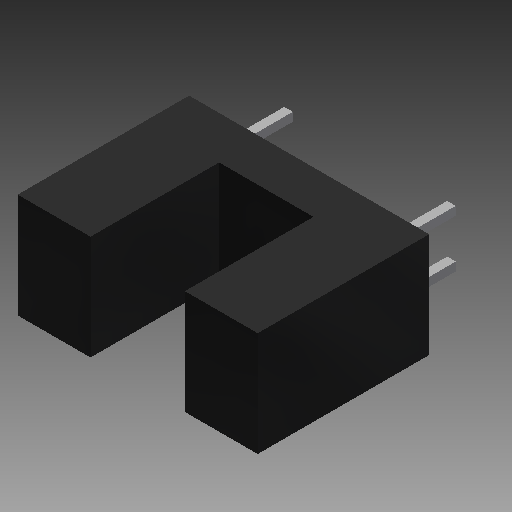
# Autodesk Inventor part: tacometer_ct
Saved by Autodesk Inventor 2019.4 (Build 234330000, 330)
## iProperties
Created: 2019-10-30
Part Number: tacometer_ct
Material: ABS Plastic
Document SubType Name: Modeling
Designer: UFABC
Density: 1 g/cm^3
Appearance: Liso - Branco
Author: UFABC
Autodesk Inventor part; units mm, degrees
ref_plane "YZ Plane" through (0, 0, 0) normal (1, 0, 0) x (0, 1, 0)
ref_plane "XZ Plane" through (0, 0, 0) normal (0, 1, 0) x (-1, 0, 0)
ref_plane "XY Plane" through (0, 0, 0) normal (0, 0, 1) x (1, 0, 0)
sketch "Sketch1" plane through (0, 0, 0) normal (0, 1, 0) x (-1, 0, 0)
  line L0 (-6.3436, 0) -> (7.6564, 0)
  line L1 (7.6564, 0) -> (7.6564, 10)
  line L2 (3.4064, 10) -> (3.4064, 2.5)
  line L3 (3.4064, 2.5) -> (-2.0936, 2.5)
  line L4 (-2.0936, 2.5) -> (-2.0936, 10)
  line L5 (-6.3436, 10) -> (-6.3436, 0)
  line L6 (-6.3436, 10) -> (-2.0936, 10)
  line L7 (3.4064, 10) -> (7.6564, 10)
  point P0 (0, 0)
  dimension "d0" = 10
  dimension "d2" = 14
  dimension "d3" = 2.5
  dimension "d24" = 4.25
  dimension "d25" = 4.25
  constraints: 16 end point, 4 parallel, 2 perpendicular, 1 collinear, 1 horizontal
  measures "d0" distance of L0.end L1.end
  measures "d2" distance of L0.start L0.end
  measures "d3" distance between parallel lines of L0 L3
  measures "d24" distance of L5.start L4.end
  measures "d25" distance of L2.start L1.end
extrude "Extrusion1" add sketch "Sketch1" along normal blind 6.1
sketch "Sketch2" plane through (6.3436, 0, 0) normal (0, 0, -1) x (-1, 0, 0)
  line L0 (0, 0) -> (0, 6.1) projected
  line L1 (2.25, 4.5071) -> (2.75, 4.5071)
  line L2 (2.75, 4.5071) -> (2.75, 4.0071)
  line L3 (2.75, 4.0071) -> (2.25, 4.0071)
  line L4 (2.25, 4.0071) -> (2.25, 4.5071)
  line L5 (2.25, 1.6957) -> (2.75, 1.6957)
  line L6 (2.75, 1.6957) -> (2.75, 1.1957)
  line L7 (2.75, 1.1957) -> (2.25, 1.1957)
  line L8 (2.25, 1.1957) -> (2.25, 1.6957)
  line L9 (11.75, 4.5071) -> (12.25, 4.5071)
  line L10 (12.25, 4.5071) -> (12.25, 4.0071)
  line L11 (11.75, 4.0071) -> (11.75, 4.5071)
  line L12 (12.25, 4.0071) -> (11.75, 4.0071)
  line L13 (11.75, 1.6957) -> (12.25, 1.6957)
  line L14 (12.25, 1.6957) -> (12.25, 1.1957)
  line L15 (11.75, 1.1957) -> (11.75, 1.6957)
  line L16 (12.25, 1.1957) -> (11.75, 1.1957)
  point P0 (6.3436, 0)
  dimension "d6" = 0.5
  dimension "d10" = 0.5
  dimension "d11" = 0.5
  dimension "d12" = 0.5
  dimension "d13" = 0.5
  dimension "d14" = 0.5
  dimension "d15" = 0.5
  dimension "d16" = 0.5
  dimension "d17" = 2.3114
  dimension "d18" = 9
  dimension "d19" = 2.25
  constraints: 32 end point, 8 parallel, 5 perpendicular, 4 collinear
  measures "d6" distance of L1.start L1.end
  measures "d10" distance of L1.end L2.end
  measures "d11" distance of L5.start L5.end
  measures "d12" distance of L5.end L6.end
  measures "d13" distance of L9.start L9.end
  measures "d14" distance of L9.end L10.end
  measures "d15" distance of L13.start L13.end
  measures "d16" distance of L13.end L14.end
  measures "d17" distance between parallel lines of L5 L3
  measures "d18" distance between parallel lines of L11 L2
  measures "d19" distance between parallel lines of L0 L4
extrude "Extrusion2" add sketch "Sketch2" along normal blind 3.8
body "Solid1"
